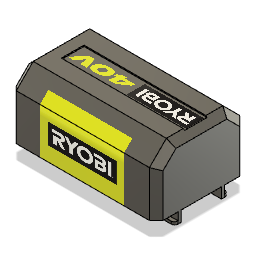
RYOBI 40V 3D Model (Autodesk Fusion 360 design; units mm, degrees)
Autodesk Fusion 360 part; units mm, degrees
sketch "Sketch1" plane through (0, 0, 0) normal (0, 1, 0) x (1, 0, 0)
  line L0 (0, 0) -> (165.1, 0)
  line L1 (165.1, 0) -> (165.1, 101.6)
  line L2 (165.1, 101.6) -> (0, 101.6)
  line L3 (0, 101.6) -> (0, 0)
  dimension "d1" = 165.1
  dimension "d2" = 101.6
  constraint horizontal L0
  constraint vertical L1
  constraint horizontal L2
  constraint vertical L3
  constraint coincident L0.start L3.end
  measures "d1" distance of L0.start L0.end
  measures "d2" distance of L0.start L2.end
extrude "Extrude1" add sketch "Sketch1" along normal blind 82.55
sketch "Sketch2" plane through (165.1, 0, 0) normal (1, 0, 0) x (0, 0, -1)
  line L0 (0, 0) -> (101.6, 0)
  line L1 (101.6, 0) -> (101.6, 82.55)
  line L2 (101.6, 82.55) -> (0, 82.55)
  line L3 (0, 82.55) -> (0, 0)
  line L4 (0, 82.55) -> (0, 63.5)
  line L5 (0, 63.5) -> (19.05, 82.55)
  line L6 (0, 82.55) -> (19.05, 82.55)
  line L7 (101.6, 82.55) -> (101.6, 63.5)
  line L8 (101.6, 63.5) -> (82.55, 82.55)
  line L9 (82.55, 82.55) -> (101.6, 82.55)
  line L10 (0, 0) -> (20.6375, 0)
  line L11 (20.6375, 0) -> (80.9625, 0)
  line L12 (80.9625, 0) -> (101.6, 0)
  line L13 (20.6375, 0) -> (20.6375, 11.938)
  line L14 (20.6375, 11.938) -> (0, 11.938)
  line L15 (0, 11.938) -> (0, 0)
  line L16 (80.9625, 0) -> (80.9625, 11.938)
  line L17 (80.9625, 11.938) -> (101.6, 11.938)
  line L18 (101.6, 0) -> (101.6, 11.938)
  line L19 (80.9625, 11.938) -> (80.9625, 0)
  dimension "d5" = 45
  dimension "d6" = 45
  dimension "d7" = 20.6375
  dimension "d8" = 60.325
  dimension "d9" = 11.938
  constraint coincident L2.end L3.start
  constraint coincident L3 L4.end
  constraint perpendicular L2 L4
  constraint coincident L2 L5.end
  constraint coincident L1.end L2.start
  constraint coincident L1 L7.end
  constraint perpendicular L2 L7
  constraint coincident L2 L8.end
  constraint perpendicular L1 L9
  constraint coincident L0.start L3.end
  constraint perpendicular L3 L10
  constraint perpendicular L1 L11
  constraint coincident L0.end L1.start
  constraint perpendicular L11 L13
  constraint coincident L3 L14.end
  constraint perpendicular L3 L14
  constraint perpendicular L0 L16
  constraint perpendicular L16 L17
  measures "d5" angle of L4 L5
  measures "d6" angle of L7 L8
  measures "d7" distance of L0.start L10.end
  measures "d8" distance of L10.end L11.end
  measures "d9" distance of L10.end L13.end
extrude "Extrude2" cut sketch "Sketch2" against normal blind 254 contours L0 L3 L10 L13 L14 L15 | L0 L1 L12 L16 L17 L18 L19 | L2 L3 L4 L5 L6 | L1 L2 L7 L8 L9
sketch "Sketch3" plane through (0, 0, 0) normal (0, -1, 0) x (1, 0, 0)
  line L0 (165.1, -20.6375) -> (0, -20.6375)
  line L1 (0, -20.6375) -> (0, -80.9625)
  line L2 (0, -80.9625) -> (165.1, -80.9625)
  line L3 (165.1, -80.9625) -> (165.1, -20.6375)
  line L4 (165.1, -20.6375) -> (165.1, -28.2575)
  line L5 (165.1, -80.9625) -> (165.1, -73.3425)
  line L6 (165.1, -28.2575) -> (152.4, -28.2575)
  line L7 (152.4, -28.2575) -> (152.4, -73.3425)
  line L8 (152.4, -73.3425) -> (165.1, -73.3425)
  line L9 (165.1, -73.3425) -> (165.1, -28.2575)
  line L10 (152.4, -50.8) -> (81.026, -50.8)
  line L11 (81.026, -50.8) -> (81.026, -35.052)
  line L12 (81.026, -50.8) -> (81.026, -66.548)
  line L13 (81.026, -35.052) -> (75.311, -35.052)
  line L14 (75.311, -35.052) -> (75.311, -66.548)
  line L15 (75.311, -66.548) -> (81.026, -66.548)
  line L16 (81.026, -66.548) -> (81.026, -35.052)
  line L17 (75.311, -50.8) -> (57.023, -50.8)
  line L18 (57.023, -50.8) -> (57.023, -31.115)
  line L19 (57.023, -50.8) -> (57.023, -70.485)
  line L20 (57.023, -70.485) -> (0, -70.485)
  line L21 (57.023, -31.115) -> (0, -31.115)
  line L22 (0, -31.115) -> (0, -70.485)
  dimension "d12" = 7.62
  dimension "d13" = 7.62
  dimension "d14" = 12.7
  dimension "d15" = 71.374
  dimension "d16" = 15.748
  dimension "d17" = 15.748
  dimension "d18" = 5.715
  dimension "d19" = 31.496
  dimension "d20" = 18.288
  dimension "d21" = 19.685
  dimension "d22" = 19.685
  constraint coincident L0.start L3.end
  constraint perpendicular L0 L4
  constraint coincident L2.end L3.start
  constraint perpendicular L2 L5
  constraint perpendicular L4 L6
  constraint perpendicular L6 L7
  constraint perpendicular L3 L8
  constraint midpoint L7 L10.start
  constraint perpendicular L7 L10
  constraint perpendicular L10 L11
  constraint perpendicular L10 L12
  constraint horizontal L13
  constraint vertical L14
  constraint horizontal L15
  constraint vertical L16
  constraint midpoint L14 L17.start
  constraint perpendicular L14 L17
  constraint perpendicular L17 L18
  constraint perpendicular L17 L19
  constraint coincident L1 L20.end
  constraint perpendicular L1 L20
  constraint coincident L1 L21.end
  constraint perpendicular L1 L21
  measures "d12" distance of L0.start L4.end
  measures "d13" distance of L2.end L5.end
  measures "d14" distance of L4.end L6.end
  measures "d15" distance of L10.start L10.end
  measures "d16" distance of L10.end L11.end
  measures "d17" distance of L10.end L12.end
  measures "d18" distance of L11.end L13.end
  measures "d19" distance of L11.end L12.end
  measures "d20" distance of L17.start L17.end
  measures "d21" distance of L17.end L18.end
  measures "d22" distance of L17.end L19.end
extrude "Extrude3" cut sketch "Sketch3" against normal up to surface (11.938 mm away) contours L3 L6 L7 L8 L9
extrude "Extrude4" add sketch "Sketch3" along normal blind 4.064 contours L11 L12 L13 L14 L15 L16
sketch "Sketch4" plane through (0, 0, -66.548) normal (0, 0, -1) x (-1, 0, 0)
  line L0 (-75.311, 0) -> (-81.026, 0)
  line L1 (-81.026, 0) -> (-81.026, -4.064)
  line L2 (-81.026, -4.064) -> (-75.311, -4.064)
  line L3 (-75.311, -4.064) -> (-75.311, 0)
  line L4 (-75.311, -4.064) -> (-81.026, 0)
  line L5 (-81.026, 0) -> (-81.026, -4.064)
  line L6 (-75.311, -4.064) -> (-81.026, -4.064)
  constraint coincident L2.end L3.start
  constraint coincident L0.end L1.start
  constraint coincident L1.end L2.start
extrude "Extrude5" cut sketch "Sketch4" against normal blind 38.1 contours L1 L2 L4 L5 L6
extrude "Extrude6" cut sketch "Sketch3" against normal blind 1.27 contours L1 L18 L19 L20 L21 L22
sketch "Sketch5" plane through (0, 0, 0) normal (-1, 0, 0) x (0, 0, 1)
  line L0 (-70.485, 0) -> (-70.485, 1.27)
  line L1 (-70.485, 1.27) -> (-31.115, 1.27)
  line L2 (-31.115, 1.27) -> (-31.115, 0)
  line L3 (-31.115, 0) -> (-20.6375, 0)
  line L4 (-20.6375, 0) -> (-20.6375, 11.938)
  line L5 (-20.6375, 11.938) -> (0, 11.938)
  line L6 (0, 11.938) -> (0, 63.5)
  line L7 (0, 63.5) -> (-19.05, 82.55)
  line L8 (-19.05, 82.55) -> (-82.55, 82.55)
  line L9 (-82.55, 82.55) -> (-101.6, 63.5)
  line L10 (-101.6, 63.5) -> (-101.6, 11.938)
  line L11 (-101.6, 11.938) -> (-80.9625, 11.938)
  line L12 (-80.9625, 11.938) -> (-80.9625, 0)
  line L13 (-80.9625, 0) -> (-70.485, 0)
  line L14 (-31.115, 1.27) -> (-70.485, 1.27)
  line L15 (-70.485, 1.27) -> (-70.485, 5.0232)
  line L16 (-70.485, 5.0232) -> (-31.115, 5.0232)
  line L17 (-31.115, 5.0232) -> (-31.115, 1.27)
  constraint horizontal L14
  constraint vertical L15
  constraint horizontal L16
  constraint vertical L17
  constraint coincident L1.end L2.start
extrude "Extrude7" cut sketch "Sketch5" against normal blind 1.27 contours L1 L14 L15 L16 L17
sketch "Sketch6" plane through (165.1, 0, 0) normal (1, 0, 0) x (0, 0, -1)
  line L0 (73.3425, 11.938) -> (73.3425, 0)
  line L1 (73.3425, 0) -> (80.9625, 0)
  line L2 (80.9625, 0) -> (80.9625, 11.938)
  line L3 (80.9625, 11.938) -> (101.6, 11.938)
  line L4 (101.6, 11.938) -> (101.6, 63.5)
  line L5 (101.6, 63.5) -> (82.55, 82.55)
  line L6 (82.55, 82.55) -> (19.05, 82.55)
  line L7 (19.05, 82.55) -> (0, 63.5)
  line L8 (0, 63.5) -> (0, 11.938)
  line L9 (0, 11.938) -> (20.6375, 11.938)
  line L10 (20.6375, 11.938) -> (20.6375, 0)
  line L11 (20.6375, 0) -> (28.2575, 0)
  line L12 (28.2575, 0) -> (28.2575, 11.938)
  line L13 (28.2575, 11.938) -> (73.3425, 11.938)
  line L14 (20.6375, 11.938) -> (24.7015, 11.938)
  line L15 (24.7015, 11.938) -> (24.7015, 3.048)
  line L16 (24.7015, 3.048) -> (20.6375, 3.048)
  line L17 (20.6375, 3.048) -> (20.6375, 11.938)
  line L18 (80.9625, 11.938) -> (76.8985, 11.938)
  line L19 (76.8985, 11.938) -> (76.8985, 3.048)
  line L20 (76.8985, 3.048) -> (80.9625, 3.048)
  line L21 (80.9625, 3.048) -> (80.9625, 11.938)
  dimension "d33" = 4.064
  dimension "d34" = 8.89
  dimension "d35" = 4.064
  dimension "d36" = 8.89
  constraint coincident L9.end L10.start
  constraint perpendicular L10 L14
  constraint perpendicular L14 L15
  constraint coincident L10 L16.end
  constraint perpendicular L10 L16
  constraint coincident L2.end L3.start
  constraint perpendicular L2 L18
  constraint perpendicular L18 L19
  constraint coincident L2 L20.end
  constraint perpendicular L2 L20
  measures "d33" distance of L9.end L14.end
  measures "d34" distance of L14.end L15.end
  measures "d35" distance of L2.end L18.end
  measures "d36" distance of L18.end L19.end
extrude "Extrude8" cut sketch "Sketch6" against normal blind 110.744 contours L2 L18 L19 L20 L21
extrude "Extrude9" cut sketch "Sketch6" against normal blind 110.744 contours L10 L14 L15 L16 L17
fillet "Fillet1" radius 3.81 2 edges at (165.1, 1.524, -80.9625) (165.1, 1.524, -20.6375)
sketch "Sketch7" plane through (152.4, 0, 0) normal (1, 0, 0) x (0, 0, -1)
  line L0 (73.3425, 11.938) -> (28.2575, 11.938)
  line L1 (28.2575, 11.938) -> (28.2575, 0)
  line L2 (28.2575, 0) -> (73.3425, 0)
  line L3 (73.3425, 0) -> (73.3425, 11.938)
  line L4 (73.3425, 11.938) -> (28.2575, 11.938)
  line L5 (28.2575, 11.938) -> (28.2575, 3.302)
  line L6 (28.2575, 3.302) -> (73.3425, 3.302)
  line L7 (73.3425, 3.302) -> (73.3425, 11.938)
  line L8 (73.3425, 3.302) -> (65.7225, 3.302)
  line L9 (65.7225, 3.302) -> (65.7225, 10.16)
  line L10 (65.7225, 10.16) -> (64.9605, 10.16)
  line L11 (64.9605, 10.16) -> (64.9605, 3.302)
  line L12 (64.9605, 3.302) -> (65.7225, 3.302)
  line L13 (28.2575, 3.302) -> (35.8775, 3.302)
  line L14 (35.8775, 3.302) -> (35.8775, 10.16)
  line L15 (35.8775, 10.16) -> (36.6395, 10.16)
  line L16 (36.6395, 10.16) -> (36.6395, 3.302)
  dimension "d43" = 8.636
  dimension "d44" = 7.62
  dimension "d45" = 0.762
  dimension "d46" = 7.62
  dimension "d47" = 6.858
  dimension "d48" = 0.762
  constraint horizontal L4
  constraint vertical L5
  constraint horizontal L6
  constraint vertical L7
  constraint coincident L1 L5.end
  constraint coincident L0.start L3.end
  constraint perpendicular L7 L8
  constraint perpendicular L6 L9
  constraint horizontal L10
  constraint coincident L6 L11.end
  constraint perpendicular L6 L11
  constraint perpendicular L5 L13
  constraint perpendicular L13 L14
  constraint perpendicular L14 L15
  constraint coincident L6 L16.end
  constraint perpendicular L6 L16
  measures "d43" distance of L0.start L6.end
  measures "d44" distance of L6.end L8.end
  measures "d45" distance of L9.end L10.end
  measures "d46" distance of L5.end L13.end
  measures "d47" distance of L13.end L14.end
  measures "d48" distance of L14.end L15.end
extrude "Extrude10" cut sketch "Sketch7" against normal blind 12.7 contours L0 L1 L3 L4 L5 L6 L7 L8 L9 L10 L11 L13 L14 L15 L16
sketch "Sketch8" plane through (165.1, 0, 0) normal (1, 0, 0) x (0, 0, -1)
  line L0 (24.4475, 3.048) -> (24.4475, 0)
  line L1 (24.4475, 0) -> (28.2575, 0)
  line L2 (28.2575, 0) -> (28.2575, 11.938)
  line L3 (28.2575, 11.938) -> (73.3425, 11.938)
  line L4 (73.3425, 11.938) -> (73.3425, 0)
  line L5 (73.3425, 0) -> (77.1525, 0)
  line L6 (77.1525, 0) -> (77.1525, 3.048)
  line L7 (77.1525, 3.048) -> (76.8985, 3.048)
  line L8 (76.8985, 3.048) -> (76.8985, 11.938)
  line L9 (76.8985, 11.938) -> (101.6, 11.938)
  line L10 (101.6, 11.938) -> (101.6, 63.5)
  line L11 (101.6, 63.5) -> (82.55, 82.55)
  line L12 (82.55, 82.55) -> (19.05, 82.55)
  line L13 (19.05, 82.55) -> (0, 63.5)
  line L14 (0, 63.5) -> (0, 11.938)
  line L15 (0, 11.938) -> (24.7015, 11.938)
  line L16 (24.7015, 11.938) -> (24.7015, 3.048)
  line L17 (24.7015, 3.048) -> (24.4475, 3.048)
  line L18 (50.8, 82.55) -> (63.5, 82.55)
  line L19 (50.8, 82.55) -> (38.1, 82.55)
  line L20 (38.1, 82.55) -> (38.1, 81.28)
  line L21 (38.1, 81.28) -> (63.5, 81.28)
  line L22 (63.5, 81.28) -> (63.5, 82.55)
  dimension "d51" = 1.27
  constraint midpoint L12 L18.start
  constraint coincident L12 L18.end
  constraint parallel L12 L18
  constraint coincident L12 L19.end
  constraint perpendicular L12 L20
  constraint perpendicular L20 L21
  constraint perpendicular L12 L22
  measures "d51" distance of L19.end L20.end
extrude "Extrude11" cut sketch "Sketch8" against normal blind 144.78 contours L12 L18 L19 L20 L21 L22
sketch "Sketch9" plane through (0, 81.28, 0) normal (0, 1, 0) x (-1, 0, 0)
  line L0 (-165.1, -38.1) -> (-165.1, -63.5)
  line L1 (-165.1, -63.5) -> (-20.32, -63.5)
  line L2 (-20.32, -63.5) -> (-20.32, -38.1)
  line L3 (-20.32, -38.1) -> (-165.1, -38.1)
chamfer "Chamfer2" distance 7.62 angle 45 6 edges at (165.1, 82.55, -73.025) (165.1, 73.025, -92.075) (165.1, 37.719, -101.6) (165.1, 82.55, -28.575) (165.1, 73.025, -9.525) (165.1, 37.719, 0)
chamfer "Chamfer3" distance 7.62 angle 45 5 edges at (0, 37.719, -101.6) (0, 73.025, -92.075) (0, 82.55, -50.8) (0, 73.025, -9.525) (0, 37.719, 0)
